# Autodesk Inventor part: FX8C-060S-SV_92_
Saved by Autodesk Inventor 2015 SP1 (Build 190203100, 203)
## iProperties
Created: 2015-10-19
Part Number: FX8C-060S-SV_92_
Material: Generic
Document SubType Name: Modeling
Designer: Kartikye
Density: 1 g/cm^3
Appearance: FX8C-060S-SV_92_, FX8C-060S-SV_92_
Author: Kartikye
Autodesk Inventor part; units mm, degrees
ref_plane "YZ Plane" through (0, 0, 0) normal (1, 0, 0) x (0, 1, 0)
ref_plane "XZ Plane" through (0, 0, 0) normal (0, 1, 0) x (-1, 0, 0)
ref_plane "XY Plane" through (0, 0, 0) normal (0, 0, 1) x (1, 0, 0)
sketch "FX8C-060S-SV_92_, FX8C-060S-SV_92__88" plane through (0, 0, 0) normal (0, 0, 1) x (1, 0, 0)
  line L0 (-12.3, 2.8635) -> (12.3635, 2.8635)
  line L1 (12.3635, 2.8635) -> (12.3635, -2.8635)
  line L2 (12.3635, -2.8635) -> (-12.3, -2.8635)
  line L3 (-12.3, -2.8635) -> (-12.3, 2.8635)
  constraints: 8 end point
extrude "Extrusion1" add sketch "FX8C-060S-SV_92_, FX8C-060S-SV_92__88" along normal blind 1
body "Solid1"
